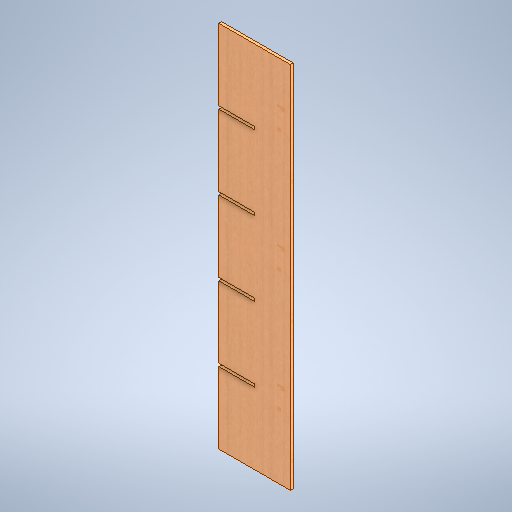
# Autodesk Inventor part: Separador
Saved by Autodesk Inventor 2025.2 (Build 292293000, 293)
## iProperties
Created: 2025-05-13
Part Number: Separador
Material: Wood (Cherry)
Document SubType Name: Modeling
Designer: USER
Density: 0.63 g/cm^3
Appearance: Cherry - Natural Low Gloss
Author: USER
Autodesk Inventor part; units mm, degrees
ref_plane "YZ Plane" through (0, 0, 0) normal (1, 0, 0) x (0, 1, 0)
ref_plane "XZ Plane" through (0, 0, 0) normal (0, 1, 0) x (-1, 0, 0)
ref_plane "XY Plane" through (0, 0, 0) normal (0, 0, 1) x (1, 0, 0)
sketch "Sketch1" plane through (0, 0, 0) normal (0, 0, 1) x (1, 0, 0)
  line L0 (0, 0) -> (150, 0)
  line L1 (150, 0) -> (150, -774)
  line L2 (150, -774) -> (0, -774)
  line L3 (0, -774) -> (0, 0)
  dimension "d0" = 150
  dimension "d1" = 774
  constraints: 8 end point, 2 parallel, 1 horizontal, 1 perpendicular
  measures "d0" distance of L1.end L2.end
  measures "d1" distance of L0.end L1.end
extrude "Extrusion1" add sketch "Sketch1" along normal blind 6
sketch "Sketch2" plane through (0, 0, 6) normal (0, 0, 1) x (1, 0, 0)
  line L0 (0, 0) -> (0, -774) projected
  line L1 (0, -150) -> (150, -150)
  line L2 (150, -774) -> (150, 0) projected
  line L3 (0, -156) -> (150, -156)
  line L4 (150, 0) -> (0, 0) projected
  line L5 (0, -306) -> (150, -306)
  line L6 (0, -312) -> (150, -312)
  line L7 (0, -462) -> (150, -462)
  line L8 (0, -468) -> (150, -468)
  line L9 (0, -618) -> (150, -618)
  line L10 (0, -624) -> (150, -624)
  line L11 (0, -774) -> (150, -774)
  line L12 (0, -780) -> (150, -780)
  line L13 (75, 0) -> (75, -774)
  line L14 (0, -774) -> (150, -774) projected
  line L15 (0, 0) -> (0, -774)
  point P0 (75, -306)
  point P1 (75, -618)
  point P2 (75, -156)
  point P3 (75, -150)
  point P4 (75, -312)
  point P5 (75, -306)
  point P6 (75, -468)
  point P7 (75, -462)
  point P8 (75, -624)
  point P9 (75, -618)
  point P10 (75, -780)
  point P11 (75, -774)
  dimension "d4" = 150
  dimension "d5" = 6
  dimension "d6" = 150
  dimension "d8" = 6
  dimension "d9" = 150
  dimension "d10" = 6
  dimension "d11" = 150
  dimension "d12" = 6
  dimension "d13" = 150
  dimension "d14" = 6
  constraints: 24 end point, 10 horizontal, 4 midpoint, 1 perpendicular, 20 other
  measures "d4" distance between parallel lines of L1 L4
  measures "d5" distance between parallel lines of L1 L3
  measures "d6" distance from line of L3 point (75, -306)
  measures "d8" distance between parallel lines of L5 L6
  measures "d9" distance between parallel lines of L7 L6
  measures "d10" distance between parallel lines of L7 L8
  measures "d11" distance from line of L8 point (75, -618)
  measures "d12" distance between parallel lines of L9 L10
  measures "d13" distance between parallel lines of L10 L11
  measures "d14" distance between parallel lines of L11 L12
extrude "Extrusion2" cut sketch "Sketch2" against normal blind 6 contours L1 L13 L3 L0 | L5 L13 L6 L0 | L7 L13 L8 L0 | L9 L13 L10 L0
body "Solid1"
